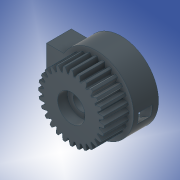
# Autodesk Inventor part: FA008
Saved by Autodesk Inventor 2017 SP1 (Build 210196100, 196)
## iProperties
Created: 2017-06-19
Part Number: FA008
Material: ABS Plastic
Document SubType Name: Modeling
Designer: Zach
Density: 1.06 g/cm^3
Appearance: CR Dark Blue
Author: Zach
Autodesk Inventor part; units mm, degrees
ref_plane "YZ Plane" through (0, 0, 0) normal (1, 0, 0) x (0, 1, 0)
ref_plane "XZ Plane" through (0, 0, 0) normal (0, 1, 0) x (-1, 0, 0)
ref_plane "XY Plane" through (0, 0, 0) normal (0, 0, 1) x (1, 0, 0)
sketch "Sketch1" plane through (0, 0, 0) normal (0, 0, 1) x (1, 0, 0)
  circle A0 centre (0, 0) radius 6.5
  circle A1 centre (0, 0) radius 22.5
  dimension "d0" = 13
  dimension "d1" = 45
  constraints: 2 centre point, 2 coincident
  measures "d0" diameter of A0
  measures "d1" diameter of A1
extrude "Extrusion1" add sketch "Sketch1" along normal blind 40
sketch "Sketch2" plane through (0, 0, 40) normal (0, 0, 1) x (1, 0, 0)
  line L0 (0, 0) -> (36.920116, 0) construction
  circle A0 centre (0, 0) radius 22.5
  arc A1 (26.410935, 0.9) -> (22.410935, 2) centre (20.471799, -12.87413) ccw
  arc A2 (26.410935, -0.9) -> (26.410935, 0.9) centre (6.431195, 0) ccw
  arc A3 (22.410935, -2) -> (26.410935, -0.9) centre (20.471799, 12.87413) ccw
  arc A4 (22.410935, -2) -> (22.410935, 2) centre (0, 0) ccw
  circle A5 centre (0, 0) radius 22.5
  arc A6 (25.548489, 6.754421) -> (21.404004, 6.936758) centre (22.823292, -7.995945) ccw
  arc A7 (25.949026, 4.999551) -> (25.548489, 6.754421) centre (6.269952, 1.431076) ccw
  arc A8 (22.294088, 3.037046) -> (25.949026, 4.999551) centre (17.093765, 17.106753) ccw
  arc A9 (22.294088, 3.037046) -> (21.404004, 6.936758) centre (0, 0) ccw
  arc A10 (23.404935, 12.270147) -> (19.323787, 11.525678) centre (24.030329, -2.71681) ccw
  arc A11 (24.185925, 10.648403) -> (23.404935, 12.270147) centre (5.794307, 2.790391) ccw
  arc A12 (21.059322, 7.921802) -> (24.185925, 10.648403) centre (12.858578, 20.481571) ccw
  arc A13 (21.059322, 7.921802) -> (19.323787, 11.525678) centre (0, 0) ccw
  arc A14 (20.08776, 17.170597) -> (16.274595, 15.536652) centre (24.032386, 2.698558) ccw
  arc A15 (21.210041, 15.7633) -> (20.08776, 17.170597) centre (5.028111, 4.009785) ccw
  arc A16 (18.768554, 12.409326) -> (21.210041, 15.7633) centre (7.978608, 22.829358) ccw
  arc A17 (18.768554, 12.409326) -> (16.274595, 15.536652) centre (0, 0) ccw
  arc A18 (15.7633, 21.210041) -> (12.409326, 18.768554) centre (22.829358, 7.978608) ccw
  arc A19 (17.170597, 20.08776) -> (15.7633, 21.210041) centre (4.009785, 5.028111) ccw
  arc A20 (15.536652, 16.274595) -> (17.170597, 20.08776) centre (2.698558, 24.032386) ccw
  arc A21 (15.536652, 16.274595) -> (12.409326, 18.768554) centre (0, 0) ccw
  arc A22 (10.648403, 24.185925) -> (7.921802, 21.059322) centre (20.481571, 12.858578) ccw
  arc A23 (12.270147, 23.404935) -> (10.648403, 24.185925) centre (2.790391, 5.794307) ccw
  arc A24 (11.525678, 19.323787) -> (12.270147, 23.404935) centre (-2.71681, 24.030329) ccw
  arc A25 (11.525678, 19.323787) -> (7.921802, 21.059322) centre (0, 0) ccw
  arc A26 (4.999551, 25.949026) -> (3.037046, 22.294088) centre (17.106753, 17.093765) ccw
  arc A27 (6.754421, 25.548489) -> (4.999551, 25.949026) centre (1.431076, 6.269952) ccw
  arc A28 (6.936758, 21.404004) -> (6.754421, 25.548489) centre (-7.995945, 22.823292) ccw
  arc A29 (6.936758, 21.404004) -> (3.037046, 22.294088) centre (0, 0) ccw
  arc A30 (-0.9, 26.410935) -> (-2, 22.410935) centre (12.87413, 20.471799) ccw
  arc A31 (0.9, 26.410935) -> (-0.9, 26.410935) centre (0, 6.431195) ccw
  arc A32 (2, 22.410935) -> (0.9, 26.410935) centre (-12.87413, 20.471799) ccw
  arc A33 (2, 22.410935) -> (-2, 22.410935) centre (0, 0) ccw
  arc A34 (-6.754421, 25.548489) -> (-6.936758, 21.404004) centre (7.995945, 22.823292) ccw
  arc A35 (-4.999551, 25.949026) -> (-6.754421, 25.548489) centre (-1.431076, 6.269952) ccw
  arc A36 (-3.037046, 22.294088) -> (-4.999551, 25.949026) centre (-17.106753, 17.093765) ccw
  arc A37 (-3.037046, 22.294088) -> (-6.936758, 21.404004) centre (0, 0) ccw
  arc A38 (-12.270147, 23.404935) -> (-11.525678, 19.323787) centre (2.71681, 24.030329) ccw
  arc A39 (-10.648403, 24.185925) -> (-12.270147, 23.404935) centre (-2.790391, 5.794307) ccw
  arc A40 (-7.921802, 21.059322) -> (-10.648403, 24.185925) centre (-20.481571, 12.858578) ccw
  arc A41 (-7.921802, 21.059322) -> (-11.525678, 19.323787) centre (0, 0) ccw
  arc A42 (-17.170597, 20.08776) -> (-15.536652, 16.274595) centre (-2.698558, 24.032386) ccw
  arc A43 (-15.7633, 21.210041) -> (-17.170597, 20.08776) centre (-4.009785, 5.028111) ccw
  arc A44 (-12.409326, 18.768554) -> (-15.7633, 21.210041) centre (-22.829358, 7.978608) ccw
  arc A45 (-12.409326, 18.768554) -> (-15.536652, 16.274595) centre (0, 0) ccw
  arc A46 (-21.210041, 15.7633) -> (-18.768554, 12.409326) centre (-7.978608, 22.829358) ccw
  arc A47 (-20.08776, 17.170597) -> (-21.210041, 15.7633) centre (-5.028111, 4.009785) ccw
  arc A48 (-16.274595, 15.536652) -> (-20.08776, 17.170597) centre (-24.032386, 2.698558) ccw
  arc A49 (-16.274595, 15.536652) -> (-18.768554, 12.409326) centre (0, 0) ccw
  arc A50 (-24.185925, 10.648403) -> (-21.059322, 7.921802) centre (-12.858578, 20.481571) ccw
  arc A51 (-23.404935, 12.270147) -> (-24.185925, 10.648403) centre (-5.794307, 2.790391) ccw
  arc A52 (-19.323787, 11.525678) -> (-23.404935, 12.270147) centre (-24.030329, -2.71681) ccw
  arc A53 (-19.323787, 11.525678) -> (-21.059322, 7.921802) centre (0, 0) ccw
  arc A54 (-25.949026, 4.999551) -> (-22.294088, 3.037046) centre (-17.093765, 17.106753) ccw
  arc A55 (-25.548489, 6.754421) -> (-25.949026, 4.999551) centre (-6.269952, 1.431076) ccw
  arc A56 (-21.404004, 6.936758) -> (-25.548489, 6.754421) centre (-22.823292, -7.995945) ccw
  arc A57 (-21.404004, 6.936758) -> (-22.294088, 3.037046) centre (0, 0) ccw
  arc A58 (-26.410935, -0.9) -> (-22.410935, -2) centre (-20.471799, 12.87413) ccw
  arc A59 (-26.410935, 0.9) -> (-26.410935, -0.9) centre (-6.431195, 0) ccw
  arc A60 (-22.410935, 2) -> (-26.410935, 0.9) centre (-20.471799, -12.87413) ccw
  arc A61 (-22.410935, 2) -> (-22.410935, -2) centre (0, 0) ccw
  arc A62 (-25.548489, -6.754421) -> (-21.404004, -6.936758) centre (-22.823292, 7.995945) ccw
  arc A63 (-25.949026, -4.999551) -> (-25.548489, -6.754421) centre (-6.269952, -1.431076) ccw
  arc A64 (-22.294088, -3.037046) -> (-25.949026, -4.999551) centre (-17.093765, -17.106753) ccw
  arc A65 (-22.294088, -3.037046) -> (-21.404004, -6.936758) centre (0, 0) ccw
  arc A66 (-23.404935, -12.270147) -> (-19.323787, -11.525678) centre (-24.030329, 2.71681) ccw
  arc A67 (-24.185925, -10.648403) -> (-23.404935, -12.270147) centre (-5.794307, -2.790391) ccw
  arc A68 (-21.059322, -7.921802) -> (-24.185925, -10.648403) centre (-12.858578, -20.481571) ccw
  arc A69 (-21.059322, -7.921802) -> (-19.323787, -11.525678) centre (0, 0) ccw
  arc A70 (-20.08776, -17.170597) -> (-16.274595, -15.536652) centre (-24.032386, -2.698558) ccw
  arc A71 (-21.210041, -15.7633) -> (-20.08776, -17.170597) centre (-5.028111, -4.009785) ccw
  arc A72 (-18.768554, -12.409326) -> (-21.210041, -15.7633) centre (-7.978608, -22.829358) ccw
  arc A73 (-18.768554, -12.409326) -> (-16.274595, -15.536652) centre (0, 0) ccw
  arc A74 (-15.7633, -21.210041) -> (-12.409326, -18.768554) centre (-22.829358, -7.978608) ccw
  arc A75 (-17.170597, -20.08776) -> (-15.7633, -21.210041) centre (-4.009785, -5.028111) ccw
  arc A76 (-15.536652, -16.274595) -> (-17.170597, -20.08776) centre (-2.698558, -24.032386) ccw
  arc A77 (-15.536652, -16.274595) -> (-12.409326, -18.768554) centre (0, 0) ccw
  arc A78 (-10.648403, -24.185925) -> (-7.921802, -21.059322) centre (-20.481571, -12.858578) ccw
  arc A79 (-12.270147, -23.404935) -> (-10.648403, -24.185925) centre (-2.790391, -5.794307) ccw
  arc A80 (-11.525678, -19.323787) -> (-12.270147, -23.404935) centre (2.71681, -24.030329) ccw
  arc A81 (-11.525678, -19.323787) -> (-7.921802, -21.059322) centre (0, 0) ccw
  arc A82 (-4.999551, -25.949026) -> (-3.037046, -22.294088) centre (-17.106753, -17.093765) ccw
  arc A83 (-6.754421, -25.548489) -> (-4.999551, -25.949026) centre (-1.431076, -6.269952) ccw
  arc A84 (-6.936758, -21.404004) -> (-6.754421, -25.548489) centre (7.995945, -22.823292) ccw
  arc A85 (-6.936758, -21.404004) -> (-3.037046, -22.294088) centre (0, 0) ccw
  arc A86 (0.9, -26.410935) -> (2, -22.410935) centre (-12.87413, -20.471799) ccw
  arc A87 (-0.9, -26.410935) -> (0.9, -26.410935) centre (0, -6.431195) ccw
  arc A88 (-2, -22.410935) -> (-0.9, -26.410935) centre (12.87413, -20.471799) ccw
  arc A89 (-2, -22.410935) -> (2, -22.410935) centre (0, 0) ccw
  arc A90 (6.754421, -25.548489) -> (6.936758, -21.404004) centre (-7.995945, -22.823292) ccw
  arc A91 (4.999551, -25.949026) -> (6.754421, -25.548489) centre (1.431076, -6.269952) ccw
  arc A92 (3.037046, -22.294088) -> (4.999551, -25.949026) centre (17.106753, -17.093765) ccw
  arc A93 (3.037046, -22.294088) -> (6.936758, -21.404004) centre (0, 0) ccw
  arc A94 (12.270147, -23.404935) -> (11.525678, -19.323787) centre (-2.71681, -24.030329) ccw
  arc A95 (10.648403, -24.185925) -> (12.270147, -23.404935) centre (2.790391, -5.794307) ccw
  arc A96 (7.921802, -21.059322) -> (10.648403, -24.185925) centre (20.481571, -12.858578) ccw
  arc A97 (7.921802, -21.059322) -> (11.525678, -19.323787) centre (0, 0) ccw
  arc A98 (17.170597, -20.08776) -> (15.536652, -16.274595) centre (2.698558, -24.032386) ccw
  arc A99 (15.7633, -21.210041) -> (17.170597, -20.08776) centre (4.009785, -5.028111) ccw
  arc A100 (12.409326, -18.768554) -> (15.7633, -21.210041) centre (22.829358, -7.978608) ccw
  arc A101 (12.409326, -18.768554) -> (15.536652, -16.274595) centre (0, 0) ccw
  arc A102 (21.210041, -15.7633) -> (18.768554, -12.409326) centre (7.978608, -22.829358) ccw
  arc A103 (20.08776, -17.170597) -> (21.210041, -15.7633) centre (5.028111, -4.009785) ccw
  arc A104 (16.274595, -15.536652) -> (20.08776, -17.170597) centre (24.032386, -2.698558) ccw
  arc A105 (16.274595, -15.536652) -> (18.768554, -12.409326) centre (0, 0) ccw
  arc A106 (24.185925, -10.648403) -> (21.059322, -7.921802) centre (12.858578, -20.481571) ccw
  arc A107 (23.404935, -12.270147) -> (24.185925, -10.648403) centre (5.794307, -2.790391) ccw
  arc A108 (19.323787, -11.525678) -> (23.404935, -12.270147) centre (24.030329, 2.71681) ccw
  arc A109 (19.323787, -11.525678) -> (21.059322, -7.921802) centre (0, 0) ccw
  arc A110 (25.949026, -4.999551) -> (22.294088, -3.037046) centre (17.093765, -17.106753) ccw
  arc A111 (25.548489, -6.754421) -> (25.949026, -4.999551) centre (6.269952, -1.431076) ccw
  arc A112 (21.404004, -6.936758) -> (25.548489, -6.754421) centre (22.823292, 7.995945) ccw
  arc A113 (21.404004, -6.936758) -> (22.294088, -3.037046) centre (0, 0) ccw
  circle A114 centre (0, 0) radius 7.737821
  circle A115 centre (0, 0) radius 6.5
  point P0 (26.431195, 0)
  point P1 (22.5, 0)
  point P2 (25.76851, 5.881494)
  point P3 (21.935878, 5.006721)
  point P4 (23.813684, 11.468066)
  point P5 (20.2718, 9.762384)
  point P6 (20.66474, 16.479581)
  point P7 (17.591208, 14.028521)
  point P8 (16.479581, 20.66474)
  point P9 (14.028521, 17.591208)
  point P10 (11.468066, 23.813684)
  point P11 (9.762384, 20.2718)
  point P12 (5.881494, 25.76851)
  point P13 (5.006721, 21.935878)
  point P14 (0, 26.431195)
  point P15 (0, 22.5)
  point P16 (-5.881494, 25.76851)
  point P17 (-5.006721, 21.935878)
  point P18 (-11.468066, 23.813684)
  point P19 (-9.762384, 20.2718)
  point P20 (-16.479581, 20.66474)
  point P21 (-14.028521, 17.591208)
  point P22 (-20.66474, 16.479581)
  point P23 (-17.591208, 14.028521)
  point P24 (-23.813684, 11.468066)
  point P25 (-20.2718, 9.762384)
  point P26 (-25.76851, 5.881494)
  point P27 (-21.935878, 5.006721)
  point P28 (-26.431195, 0)
  point P29 (-22.5, 0)
  point P30 (-25.76851, -5.881494)
  point P31 (-21.935878, -5.006721)
  point P32 (-23.813684, -11.468066)
  point P33 (-20.2718, -9.762384)
  point P34 (-20.66474, -16.479581)
  point P35 (-17.591208, -14.028521)
  point P36 (-16.479581, -20.66474)
  point P37 (-14.028521, -17.591208)
  point P38 (-11.468066, -23.813684)
  point P39 (-9.762384, -20.2718)
  point P40 (-5.881494, -25.76851)
  point P41 (-5.006721, -21.935878)
  point P42 (0, -26.431195)
  point P43 (0, -22.5)
  point P44 (5.881494, -25.76851)
  point P45 (5.006721, -21.935878)
  point P46 (11.468066, -23.813684)
  point P47 (9.762384, -20.2718)
  point P48 (16.479581, -20.66474)
  point P49 (14.028521, -17.591208)
  point P50 (20.66474, -16.479581)
  point P51 (17.591208, -14.028521)
  point P52 (23.813684, -11.468066)
  point P53 (20.2718, -9.762384)
  point P54 (25.76851, -5.881494)
  point P55 (21.935878, -5.006721)
  dimension "d4" = 15
  dimension "d5" = 4
  dimension "d6" = 1.8
  dimension "d7" = 20
  dimension "d8" = 2
  dimension "d9" = 15
  dimension "d12" = 360
  constraints: 228 point on circle, 113 centre point, 2 end point, 2 point on line, 1 coincident, 1 concentric, 1 horizontal, 1 vertical alignment, 395 other
  measures "d4" radius of A1
  measures "d5" horizontal distance of A1.start A0.start
  measures "d6" distance of A1.start A2.start
  measures "d7" radius of A2
  measures "d8" vertical distance of point (26.431, 0) A0.start
  measures "d9" radius of A3
extrude "Extrusion3" add sketch "Sketch2" against normal blind 20 contours A0 | A0 A1 A2 A3 | A0 A6 A7 A8 | A110 A111 A112 A0 | A0 A10 A11 A12 | A106 A107 A108 A0 | A0 A14 A15 A16 | A102 A103 A104 A0 | A0 A18 A19 A20 | A98 A99 A100 A0 | A0 A22 A23 A24 | A94 A95 A96 A0 | A0 A26 A27 A28 | A90 A91 A92 A0 | A0 A30 A31 A32 | A86 A87 A88 A0 | A0 A34 A35 A36 | A82 A83 A84 A0 | A0 A38 A39 A40 | A78 A79 A80 A0 | A0 A42 A43 A44 | A74 A75 A76 A0 | A0 A46 A47 A48 | A70 A71 A72 A0 | A0 A50 A51 A52 | A66 A67 A68 A0 | A0 A54 A55 A56 | A62 A63 A64 A0 | A0 A58 A59 A60
sketch "Sketch3" plane through (0, 0, 0) normal (0, 0, -1) x (-1, 0, 0)
  line L0 (0, 15) -> (40, 15) construction
  line L1 (40, 15) -> (40, -15) construction
  line L2 (40, -15) -> (0, -15) construction
  line L3 (0, -15) -> (0, 15) construction
  line L4 (0, 15) -> (40, 15)
  line L5 (40, 15) -> (40, -15)
  line L6 (40, -15) -> (0, -15)
  line L7 (0, -15) -> (0, -6.5)
  circle A0 centre (0, 0) radius 6.5 projected
  line L8 (0, 15) -> (0, 6.5)
  arc A1 (0, -6.5) -> (0, 6.5) centre (0, 0) ccw
  dimension "d18" = 40
  dimension "d19" = 30
  constraints: 18 end point, 5 equal length, 4 point on circle, 2 concentric, 2 point on line, 1 centre point, 1 coincident, 1 horizontal, 1 midpoint, 1 perpendicular
  measures "d18" distance of L1.end L2.end
  measures "d19" distance of L0.end L1.end
sketch "Sketch3 outline for Extrusion4" plane through (0, 0, 0) normal (0, 0, -1) x (-1, 0, 0)
  line L0 (40, 15) -> (0, 15)
  line L1 (40, -15) -> (40, 15)
  line L2 (0, -15) -> (40, -15)
  line L3 (0, -6.5) -> (0, -15)
  arc A0 (0, 6.5) -> (0, -6.5) centre (0, 0) cw
  line L4 (0, 15) -> (0, 6.5)
extrude "Extrusion4" add sketch "Sketch3 outline for Extrusion4" against normal blind 20
sketch "Sketch4" plane through (0, 0, 0) normal (0, 0, -1) x (-1, 0, 0)
  circle A0 centre (0, 0) radius 30
  circle A1 centre (0, 0) radius 6.5 projected
  dimension "d22" = 60
  constraints: 1 centre point, 1 coincident
  measures "d22" diameter of A0
extrude "Extrusion5" add sketch "Sketch4" against normal blind 20
sketch "Sketch5" plane through (-40, -15, 0) normal (-1, 0, 0) x (0, 0, 1)
  line L0 (0, 30) -> (20, 30) projected
  circle A0 centre (10, 27.7) radius 1
  circle A1 centre (10, 2.3) radius 1
  line L1 (10, 27.7) -> (10, 2.3) construction
  line L2 (20, 30) -> (20, 0) construction
  line L3 (16, 26) -> (4, 26)
  line L4 (4, 26) -> (4, 4)
  line L5 (4, 4) -> (16, 4)
  line L6 (16, 4) -> (16, 26)
  point P0 (0, 15)
  point P1 (10, 30)
  point P2 (10, 30)
  point P3 (20, 15)
  point P4 (10, 15)
  point P5 (10, 30)
  point P6 (16, 15)
  point P7 (10, 26)
  point P8 (10, 30)
  dimension "d25" = 2
  dimension "d26" = 2
  dimension "d27" = 25.4
  dimension "d28" = 22
  dimension "d29" = 12
  constraints: 10 end point, 8 midpoint, 2 centre point, 2 horizontal alignment, 2 parallel, 2 vertical alignment, 1 coincident, 1 horizontal, 1 perpendicular, 1 vertical
  measures "d25" diameter of A0
  measures "d26" diameter of A1
  measures "d27" distance of L1.end L1.start
  measures "d28" distance of L5.end L3.start
  measures "d29" distance between parallel lines of L4 L6
extrude "Extrusion6" cut sketch "Sketch5" against normal blind 20
sketch "Sketch6" plane through (-40, -11, 16) normal (0, 0, -1) x (-1, 0, 0)
  line L0 (0, 22) -> (0, 0)
  line L1 (0, 22) -> (-20, 22)
  line L2 (-20, 22) -> (-20, 0)
  line L3 (0, 0) -> (-20, 0)
  line L4 (-20, 5) -> (-15, 0)
  line L5 (-40, 11) -> (-40, -49) construction
  line L6 (-40, 11) -> (20, 11) construction
  line L7 (-20, 5) -> (-40, -6.547005)
  line L8 (-20, 5) -> (3.094011, 5) construction
  line L9 (-15, 0) -> (-40, -14.433757)
  line L10 (-15, 0) -> (13.867513, 0) construction
  line L11 (-40, -6.547005) -> (-69.999141, 10.773007)
  line L12 (-40, -14.433757) -> (-68.652081, 2.10853)
  arc A0 (-69.999141, 10.773007) -> (-68.652081, 2.10853) centre (-40, 11) ccw
  arc A1 (-14.019238, 26) -> (-14.019238, -4) centre (-40, 11) ccw construction
  dimension "d32" = 5
  dimension "d33" = 45
  dimension "d34" = 60
  dimension "d35" = 90
  dimension "d36" = 150
  dimension "d37" = 150
  dimension "d38" = 120
  constraints: 18 end point, 4 point on line, 3 equal length, 3 horizontal, 2 point on circle, 1 centre point, 1 parallel, 1 vertical
  measures "d32" distance of L2.end L4.start
  measures "d33" angle of L4 L2
  measures "d34" distance of L5.start L5.end
  measures "d35" angle of L5 L6
  measures "d36" angle of L7 L8
  measures "d37" angle of L9 L10
  measures "d38" angle of L5 L12
extrude "Extrusion7" cut sketch "Sketch6" along normal through all contours L9 L12 A0 L11 L7 L2 L3 | L3 L2 L4
sketch "Sketch8" plane through (0, 0, 0) normal (0, 0, -1) x (-1, 0, 0)
  arc A0 (25.980762, 15) -> (-29.999141, -0.226993) centre (0, 0) ccw
  line L0 (-29.999141, -0.226993) -> (0, -17.547005)
  line L1 (0, -17.547005) -> (20, -6)
  line L2 (20, -6) -> (25, -11)
  line L3 (25, -11) -> (0, -25.433757)
  line L4 (0, -25.433757) -> (-28.652081, -8.89147)
  arc A1 (-28.652081, -8.89147) -> (25.980762, -15) centre (0, 0) ccw
  line L5 (25.980762, -15) -> (40, -15)
  line L6 (40, -15) -> (40, 15)
  line L7 (40, 15) -> (25.980762, 15)
  arc A2 (25.980762, 15) -> (-29.999141, -0.226993) centre (0, 0) ccw
  circle A3 centre (0, 0) radius 6.5
  arc A4 (-29.999141, -0.226993) -> (-28.652081, -8.89147) centre (0, 0) ccw
  constraints: 2 point on circle, 1 centre point
extrude "Extrusion8" add sketch "Sketch8" against normal blind 5 contours L0 L1 L2 L3 L4 A4
sketch "Sketch9" plane through (0, 0, 0) normal (0, 0, -1) x (-1, 0, 0)
  line L0 (-28.652081, -8.89147) -> (0, -25.433757)
  line L1 (0, -17.547005) -> (-29.999141, -0.226993)
  line L2 (20, -6) -> (0, -17.547005)
  line L3 (0, -25.433757) -> (25, -11)
  line L4 (40, -11) -> (25, -11)
  line L5 (20, -6) -> (20, 11)
  line L6 (40, 11) -> (20, 11)
  line L7 (-20, -6) -> (-20, -13.886751)
  line L8 (-8, -20.814955) -> (-8, -12.928203)
  point P0 (0, 0)
  dimension "d43" = 12
  constraints: 4 end point, 4 point on line, 1 horizontal alignment, 1 parallel, 1 vertical
  measures "d43" distance between parallel lines of L8 L7
extrude "Extrusion9" cut sketch "Sketch9" against normal blind 10
sketch "Sketch10" plane through (0, 0, 40) normal (0, 0, 1) x (1, 0, 0)
  circle A0 centre (0, 0) radius 11
  dimension "d46" = 22
  constraints: 1 centre point, 1 coincident
  measures "d46" diameter of A0
extrude "Extrusion10" cut sketch "Sketch10" against normal blind 8
sketch "Sketch11" plane through (0, 0, 0) normal (0, 0, -1) x (-1, 0, 0)
  circle A0 centre (0, 0) radius 11
  dimension "d49" = 22
  constraints: 1 centre point, 1 coincident
  measures "d49" diameter of A0
extrude "Extrusion11" cut sketch "Sketch11" against normal blind 8
body "Solid1"
